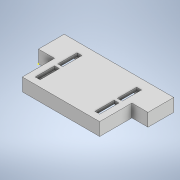
# Autodesk Inventor part: led-reed-compartment
Saved by Autodesk Inventor 2021 (Build 250183000, 183)
## iProperties
Created: 2021-01-19
Part Number: led-reed-compartment
Material: Generic
Document SubType Name: Modeling
Designer: Luke Kamols
Density: 1 g/cm^3
Appearance: Default
Author: Luke Kamols
Autodesk Inventor part; units mm, degrees
ref_plane "YZ Plane" through (0, 0, 0) normal (1, 0, 0) x (0, 1, 0)
ref_plane "XZ Plane" through (0, 0, 0) normal (0, 1, 0) x (-1, 0, 0)
ref_plane "XY Plane" through (0, 0, 0) normal (0, 0, 1) x (1, 0, 0)
sketch "Sketch1" plane through (0, 0, 0) normal (0, 1, 0) x (-1, 0, 0)
  line L0 (-34, 0) -> (-34, -8)
  line L1 (-34, -8) -> (0, -8)
  line L2 (0, -8) -> (0, 0)
  line L3 (0, 0) -> (0, -1)
  line L4 (-33, -1) -> (-33, -7)
  line L5 (-33, -7) -> (-1, -7)
  line L6 (-1, -7) -> (-1, -1)
  line L7 (-5, 0) -> (-5, 10)
  line L8 (-5, 10) -> (-29, 10)
  line L9 (-29, 10) -> (-29, 0)
  line L10 (-29, 10) -> (-29, 9)
  line L11 (-1, -1) -> (-5, -1)
  line L12 (-29, -1) -> (-33, -1)
  line L13 (-29, -1) -> (-28, -1)
  line L14 (0, 0) -> (-5, 0)
  line L15 (-34, 0) -> (-29, 0)
  line L16 (-28, -1) -> (-28, 9)
  line L17 (-28, 9) -> (-6, 9)
  line L18 (-6, 9) -> (-6, -1)
  line L19 (-6, -1) -> (-5, -1)
  line L20 (0, 0) -> (-5, 0)
  dimension "d0" = 34
  dimension "d1" = 8
  dimension "d4" = 32
  dimension "d5" = 6
  dimension "d9" = 24
  dimension "d17" = 10
  dimension "d18" = 22
  constraints: 42 end point, 6 parallel, 6 perpendicular, 4 horizontal, 2 point on line, 1 collinear
  measures "d0" distance of L1.end L0.end
  measures "d1" distance of L0.end L0.start
  measures "d4" distance of L5.end L4.end
  measures "d5" distance of L4.end L4.start
  measures "d9" distance of L7.end L8.end
  measures "d17" distance of L13.end L16.end
  measures "d18" distance of L16.end L17.end
extrude "Extrusion1" add sketch "Sketch1" along normal blind 3
sketch "Sketch2" plane through (0, 3, 0) normal (0, 1, 0) x (1, 0, 0)
  line L0 (0, 8) -> (0, 0) projected
  line L1 (34, 8) -> (0, 8) projected
  line L2 (34, 0) -> (34, 8) projected
  line L3 (29, 0) -> (34, 0) projected
  line L4 (29, -10) -> (29, 0) projected
  line L5 (5, -10) -> (29, -10) projected
  line L6 (5, 0) -> (5, -10) projected
  line L7 (0, 0) -> (5, 0) projected
extrude "Extrusion2" add sketch "Sketch2" along normal blind 1
sketch "Sketch3" plane through (0, 3, 0) normal (0, -1, 0) x (1, 0, 0)
  line L0 (33, -7) -> (33, -1) projected
  line L1 (33, -1) -> (28, -1) projected
  line L2 (28, -1) -> (28, 9) projected
  line L3 (28, 9) -> (6, 9) projected
  line L4 (6, 9) -> (6, -1) projected
  line L5 (6, -1) -> (1, -1) projected
  line L6 (1, -1) -> (1, -7) projected
  line L7 (1, -7) -> (33, -7) projected
  line L8 (28, 9) -> (6, 9) projected
  line L9 (6, 9) -> (6, 8)
  line L10 (6, 9) -> (6, -1) projected
  line L11 (6, 8) -> (7, 8)
  line L12 (7, 8) -> (8.5, 8)
  line L13 (8.5, 8) -> (8.5, 2)
  line L14 (8.5, 2) -> (7, 2)
  line L15 (7, 2) -> (7, 8)
  line L16 (7, 2) -> (7, 1)
  line L17 (7, 1) -> (8.5, 1)
  line L18 (8.5, 1) -> (8.5, -5)
  line L19 (8.5, -5) -> (7, -5)
  line L20 (7, -5) -> (7, 1)
  line L21 (28, -1) -> (28, 9) projected
  line L22 (28, 9) -> (28, 8)
  line L23 (28, 8) -> (27, 8)
  line L24 (27, 8) -> (25.5, 8)
  line L25 (25.5, 8) -> (25.5, 2)
  line L26 (25.5, 2) -> (27, 2)
  line L27 (27, 2) -> (27, 8)
  line L28 (27, 2) -> (27, 1)
  line L29 (27, 1) -> (25.5, 1)
  line L30 (25.5, 1) -> (25.5, -5)
  line L31 (25.5, -5) -> (27, -5)
  line L32 (27, -5) -> (27, 1)
  point P0 (0, 0)
  dimension "d23" = 1
  dimension "d24" = 1
  dimension "d26" = 1.5
  dimension "d27" = 6
  dimension "d28" = 1
  dimension "d29" = 1.5
  dimension "d30" = 6
  dimension "d31" = 1
  dimension "d32" = 1
  dimension "d33" = 1.5
  dimension "d34" = 6
  dimension "d35" = 1
  constraints: 44 end point, 8 parallel, 6 perpendicular, 4 horizontal, 2 point on line, 2 vertical
  measures "d23" distance of L3.end L9.end
  measures "d24" distance of L9.end L11.end
  measures "d26" distance of L13.end L14.end
  measures "d27" distance of L12.end L13.end
  measures "d28" distance of L14.end L16.end
  measures "d29" distance of L18.end L19.end
  measures "d30" distance of L17.end L18.end
  measures "d31" distance of L2.end L22.end
  measures "d32" distance of L22.end L23.end
  measures "d33" distance of L26.end L25.end
  measures "d34" distance of L25.end L24.end
  measures "d35" distance of L26.end L28.end
extrude "Extrusion3" cut sketch "Sketch3" against normal blind 1 contours L32 L31 L30 L29 | L27 L26 L25 L24 | L17 L18 L19 L20 | L12 L13 L14 L15
sketch "Sketch4" plane through (0, 0, 0) normal (0, -1, 0) x (1, 0, 0)
  point P0 (0, 0)
body "Solid1"
